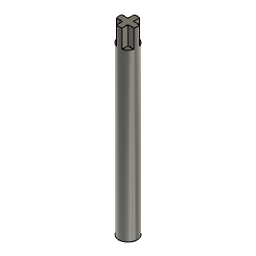
Encaixe v5 (Autodesk Fusion 360 design; units mm, degrees)
Autodesk Fusion 360 part; units mm, degrees
sketch "Sketch1" plane through (0, 0, 0) normal (0, 0, 1) x (1, 0, 0)
  circle A0 centre (0, 0) radius 10
  dimension "d1" = 20
  constraint coincident A0.centre origin
  measures "d1" diameter of A0
extrude "Extrude1" add sketch "Sketch1" along normal blind 5
sketch "Sketch2" plane through (0, 0, 5) normal (0, 0, 1) x (-1, 0, 0)
  circle A0 centre (0, 0) radius 10
  line L0 (-3, -3) -> (-3, -9.5394)
  line L1 (3, 3) -> (3, 9.5394)
  line L2 (-3, 3) -> (-3, 9.5394)
  line L3 (3, -3) -> (3, -9.5394)
  line L4 (-3, 3) -> (-9.5394, 3)
  line L5 (3, 3) -> (9.5394, 3)
  line L6 (3, -3) -> (9.5394, -3)
  line L7 (-3, -3) -> (-9.5394, -3)
  constraint coincident A0 L0.end
  constraint coincident A0 L4.end
  constraint perpendicular L2 L4
  constraint coincident A0 L3.end
  constraint coincident A0 L5.end
  constraint coincident A0 L1.end
  constraint coincident A0 L2.end
  constraint perpendicular L1 L5
  constraint coincident A0 L6.end
  constraint coincident A0 L7.end
extrude "Extrude2" add sketch "Sketch2" along normal blind 194.9 contours A0 L0 L1 L2 L3 L4 L5 L6 L7
sketch "Sketch3" plane through (0, 0, 0) normal (0, 0, -1) x (1, 0, 0)
  circle A0 centre (0, 0) radius 10
  circle A1 centre (0, 0) radius 2.5
  dimension "d14" = 5
  constraint coincident A0.centre A1.centre
  measures "d14" diameter of A1
extrude "Extrude3" cut sketch "Sketch3" against normal blind 17 contours A1
extrude "Extrude4" add 4 faces at (5.7029, 5.7029, 5) (-5.7029, 5.7029, 5) (5.7029, -5.7029, 5) (-5.7029, -5.7029, 5) along direction (0, 0, 1) blind 175
equation "d12 = 196 mm - 5 mm + 3.9 mm"
equation "d17 = 195.00 mm - 20 mm"
